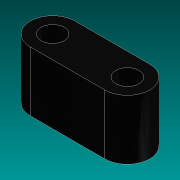
# Autodesk Inventor part: 胴体_サブフレーム_1_8
Saved by Autodesk Inventor 2015 (Build 190159000, 159)
## iProperties
Created: 2016-05-19
Part Number: 胴体_サブフレーム_1_8
Material: アセタール樹脂、黒
Document SubType Name: Modeling
Designer: hiroaki
Density: 1.425 g/cm^3
Appearance: 滑らか - 黒
Mass: 0.83424 g
Surface Area: 6.12977 cm^2
Volume: 0.585432 cm^3
Author: hiroaki
Autodesk Inventor part; units mm, degrees
ref_plane "YZ Plane" through (0, 0, 0) normal (1, 0, 0) x (0, 1, 0)
ref_plane "XZ Plane" through (0, 0, 0) normal (0, 1, 0) x (-1, 0, 0)
ref_plane "XY Plane" through (0, 0, 0) normal (0, 0, 1) x (1, 0, 0)
sketch "スケッチ1" plane through (0, 0, 0) normal (0, 0, 1) x (1, 0, 0)
  circle A0 centre (-5, 0) radius 1.55
  line L0 (0, 0) -> (-5, 0) construction
  line L1 (0, 0) -> (5, 0) construction
  circle A1 centre (5, 0) radius 1.55
  line L2 (-5, 3) -> (5, 3)
  arc A2 (-5, 3) -> (-5, -3) centre (-5, 0) ccw
  line L3 (-5, -3) -> (5, -3)
  arc A3 (5, -3) -> (5, 3) centre (5, 0) ccw
  dimension "d0" = 5
  dimension "d1" = 3.1
  dimension "d2" = 3
  constraints: 8 end point, 4 centre point, 4 horizontal, 4 point on circle, 3 coincident, 2 equal length, 2 equal radius, 1 tangent
  measures "d0" distance of L0.start L0.end
  measures "d1" diameter of A0
  measures "d2" radius of A2
extrude "押し出し1" add sketch "スケッチ1" along normal blind 8
